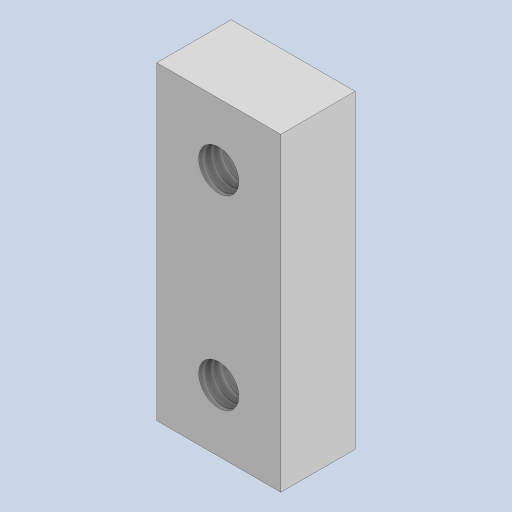
# Autodesk Inventor part: Flange attach block
Saved by Autodesk Inventor 2023.4 (Build 274418000, 418)
## iProperties
Created: 2024-02-05
Part Number: Flange attach block
Material: Generic
Document SubType Name: Modeling
Designer: PalumaCMM
Density: 1 g/cm^3
Appearance: Default
Author: PalumaCMM
Autodesk Inventor part; units mm, degrees
ref_plane "YZ Plane" through (0, 0, 0) normal (1, 0, 0) x (0, 1, 0)
ref_plane "XZ Plane" through (0, 0, 0) normal (0, 1, 0) x (-1, 0, 0)
ref_plane "XY Plane" through (0, 0, 0) normal (0, 0, 1) x (1, 0, 0)
sketch "Sketch1" plane through (0, 0, 0) normal (0, 0, 1) x (1, 0, 0)
  line L0 (0, 0) -> (10, 0)
  line L1 (10, 0) -> (10, 25)
  line L2 (10, 25) -> (0, 25)
  line L3 (0, 25) -> (0, 0)
  dimension "d0" = 10
  dimension "d1" = 25
  constraints: 8 end point, 2 parallel, 1 horizontal, 1 perpendicular
  measures "d0" distance of L2.end L1.end
  measures "d1" distance of L1.end L0.end
extrude "Extrusion1" add sketch "Sketch1" along normal blind 6
sketch "Sketch2" plane through (0, 0, 6) normal (0, 0, 1) x (1, 0, 0)
  line L0 (10, 0) -> (10, 25) construction
  line L1 (10, 25) -> (0, 25) construction
  line L2 (0, 25) -> (0, 0) construction
  line L3 (0, 0) -> (10, 0) construction
  point P0 (5, 20)
  point P1 (5, 5)
  dimension "d4" = 5
  dimension "d5" = 10
  dimension "d6" = 5
  dimension "d7" = 5
  dimension "d15" = 15
  measures "d4" distance from line of L1 point (5, 20)
  measures "d5" distance of L0.end L1.end
  measures "d6" distance from line of L2 point (5, 5)
  measures "d7" distance from line of L2 point (5, 20)
  measures "d15" distance of point (5, 5) point (5, 20)
hole "Hole1" at (5, 20, 6) at (5, 5, 6) direction (0, 0, -1) diameter 3.242 end through all thread size "M4x0.7" class "6H" standard "ISO Metric profile"
equation "\"d6\" = 0.5 * d5"
equation "\"d7\" = d6"
body "Solid1"
